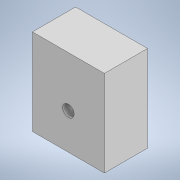
# Autodesk Inventor part: Pin Block
Saved by Autodesk Inventor 2020.4 (Build 244396000, 396)
## iProperties
Created: 2022-04-16
Part Number: Pin Block
Material: Generic
Document SubType Name: Modeling
Designer: Gurkin
Density: 1 g/cm^3
Appearance: Default
Author: Gurkin
Autodesk Inventor part; units mm, degrees
ref_plane "YZ Plane" through (0, 0, 0) normal (1, 0, 0) x (0, 1, 0)
ref_plane "XZ Plane" through (0, 0, 0) normal (0, 1, 0) x (-1, 0, 0)
ref_plane "XY Plane" through (0, 0, 0) normal (0, 0, 1) x (1, 0, 0)
sketch "Sketch1" plane through (0, 0, 0) normal (0, 0, 1) x (1, 0, 0)
  line L0 (-36, 88) -> (64, 88)
  line L1 (64, 88) -> (64, -32)
  line L2 (64, -32) -> (-36, -32)
  line L3 (-36, -32) -> (-36, 88)
  point P0 (0, 0)
  dimension "d0" = 100
  dimension "d1" = 120
  constraints: 8 end point, 2 parallel, 1 horizontal, 1 perpendicular
  measures "d0" distance between parallel lines of L1 L3
  measures "d1" distance between parallel lines of L2 L0
extrude "Extrusion1" add sketch "Sketch1" along normal blind 60
sketch "Sketch2" plane through (0, 0, 60) normal (0, 0, 1) x (1, 0, 0)
  circle A0 centre (14, 18) radius 8
  line L0 (64, 88) -> (-36, 88) projected
  line L1 (64, -32) -> (64, 88) projected
  line L2 (-36, -32) -> (64, -32) projected
  point P0 (0, 0)
  dimension "d4" = 16
  dimension "d6" = 50
  dimension "d7" = 50
  constraints: 1 centre point
  measures "d4" diameter of A0
  measures "d6" distance from line of L1 A0.centre
  measures "d7" distance from line of L2 A0.centre
extrude "Extrusion2" cut sketch "Sketch2" against normal through all
body "Solid1"
